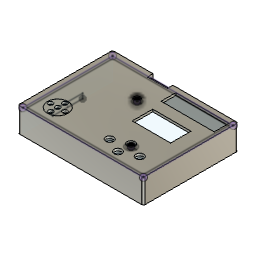
SmartDiskII 3D Case board v7 (Autodesk Fusion 360 design; units mm, degrees)
Autodesk Fusion 360 part; units mm, degrees
note: some values were not read from the file. Chosen so that the rebuilt part matches the saved one: which bodies a step acts on; which face or edge a step refers to. Set by a fixed rule: which sketch regions a step uses.
sketch "Sketch1" plane through (0, 0, 0) normal (0, 0, 1) x (1, 0, 0)
  line L0 (0, 0) -> (76.3, 0)
  line L1 (76.3, 0) -> (76.3, 56.8)
  line L2 (76.3, 56.8) -> (0, 56.8)
  line L3 (0, 56.8) -> (0, 0)
  line L4 (77.8, 58.3) -> (-1.5, 58.3)
  line L5 (-1.5, 58.3) -> (-1.5, -1.5)
  line L6 (-1.5, -1.5) -> (77.8, -1.5)
  line L7 (77.8, -1.5) -> (77.8, 58.3)
  line L8 (2.9, 56.8) -> (2.9, 58.3)
  line L9 (17.8, 56.8) -> (17.8, 58.3)
  line L10 (25.6, 56.8) -> (25.6, 58.3)
  line L11 (35.2, 58.3) -> (35.2, 56.8)
  line L12 (75.3, 58.3) -> (75.3, 56.8)
  line L13 (42.6, 58.3) -> (42.6, 56.8)
  line L14 (43.4, 38.8) -> (67.6, 38.8)
  line L15 (67.6, 38.8) -> (67.6, 25.9)
  line L16 (67.6, 25.9) -> (43.4, 25.9)
  line L17 (43.4, 25.9) -> (43.4, 38.8)
  circle A0 centre (65.2, 8.8) radius 2.5
  circle A1 centre (46.2, 8.8) radius 2.5
  circle A2 centre (55.6, 4.6) radius 2.5
  circle A3 centre (55.6, 12.9) radius 2.5
  line L18 (41.7, 55.2) -> (75.3, 55.2)
  line L19 (75.3, 55.2) -> (75.3, 45.8)
  line L20 (75.3, 45.8) -> (41.7, 45.8)
  line L21 (41.7, 45.8) -> (41.7, 55.2)
  line L22 (25.6, 56.8) -> (35.2, 56.8)
  line L23 (35.2, 56.8) -> (35.2, 47.1)
  line L24 (35.2, 47.1) -> (25.6, 47.1)
  line L25 (25.6, 47.1) -> (25.6, 56.8)
  line L26 (25.6, 42.9) -> (35.2, 42.9)
  line L27 (35.2, 42.9) -> (35.2, 36.4)
  line L28 (35.2, 36.4) -> (25.6, 36.4)
  line L29 (25.6, 36.4) -> (25.6, 42.9)
  circle A4 centre (12.4, 9.7) radius 6.5
  line L30 (25.6, 16.35) -> (30.6, 16.35)
  line L31 (30.6, 16.35) -> (30.6, 9.85)
  line L32 (30.6, 9.85) -> (25.6, 9.85)
  line L33 (25.6, 9.85) -> (25.6, 16.35)
  circle A5 centre (12, 20.2) radius 2.25
  circle A6 centre (12.4, 37.5) radius 2.25
  circle A7 centre (72.3819, 43.55) radius 1.75
  circle A8 centre (3.8963, 4.2747) radius 2.5
  circle A9 centre (72.3819, 8.8) radius 2.5
  line L34 (47.4, 40.3) -> (63.6, 40.3)
  line L35 (63.6, 40.3) -> (63.6, 44.3)
  line L36 (63.6, 44.3) -> (47.4, 44.3)
  line L37 (47.4, 44.3) -> (47.4, 40.3)
  line L38 (24.1, 58.3) -> (36.7, 58.3)
  line L39 (36.7, 58.3) -> (36.7, 56.8)
  line L40 (36.7, 56.8) -> (24.1, 56.8)
  line L41 (24.1, 56.8) -> (24.1, 58.3)
  line L42 (30.1, 42.9) -> (30.1, 36.4)
  line L43 (30.1, 36.4) -> (35.2, 42.9) construction
  line L44 (30.1, 42.9) -> (35.2, 36.4) construction
  circle A10 centre (32.65, 39.65) radius 2
  circle A11 centre (55.6, 12.9) radius 3.4
  circle A12 centre (55.6, 12.9) radius 4.15
  circle A13 centre (55.6, 4.6) radius 3.4
  circle A14 centre (55.6, 4.6) radius 4.15
  circle A15 centre (46.2, 8.8) radius 3.4
  circle A16 centre (46.2, 8.8) radius 4.15
  circle A17 centre (65.2, 8.8) radius 3.4
  circle A18 centre (65.2, 8.8) radius 4.15
  circle A19 centre (32.65, 39.65) radius 2.65
  circle A20 centre (32.65, 39.65) radius 3.4
  line L45 (12.4, 9.7) -> (12.4, 16.2) construction
  line L46 (12.4, 9.7) -> (18.9, 9.7) construction
  line L47 (12.4, 9.7) -> (12.4, 3.2) construction
  line L48 (12.4, 9.7) -> (5.9, 9.7) construction
  circle A21 centre (12.4, 9.7) radius 1.5
  circle A22 centre (12.4, 5.2) radius 1.5
  circle A23 centre (7.9, 9.7) radius 1.5
  circle A24 centre (16.9, 9.7) radius 1.5
  circle A25 centre (12.4, 14.2) radius 1.5
  dimension "d5" = 76.3
  dimension "d6" = 56.8
  dimension "d8" = 1.5
  dimension "d9" = 2.9
  dimension "d10" = 17.8
  dimension "d11" = 25.6
  dimension "d12" = 35.2
  dimension "d13" = 75.3
  dimension "d14" = 42.6
  dimension "d15" = 8.7
  dimension "d16" = 24.2
  dimension "d17" = 12.9
  dimension "d18" = 25.9
  dimension "d19" = 5
  dimension "d20" = 8.8
  dimension "d21" = 11.1
  dimension "d22" = 5
  dimension "d23" = 30.1
  dimension "d24" = 5
  dimension "d25" = 4.6
  dimension "d26" = 20.7
  dimension "d27" = 5
  dimension "d28" = 12.9
  dimension "d39" = 9.4
  dimension "d40" = 1.6
  dimension "d43" = 8.8
  dimension "d44" = 1
  dimension "d45" = 33.6
  dimension "d46" = 20.7
  dimension "d47" = 9.7
  dimension "d48" = 6.5
  dimension "d50" = 13.9
  dimension "d53" = 13
  dimension "d54" = 12.4
  dimension "d55" = 9.7
  dimension "d58" = 9.85
  dimension "d59" = 6.5
  dimension "d60" = 5
  dimension "d67" = 4.5
  dimension "d68" = 4.5
  dimension "d69" = 19.3
  dimension "d70" = 20.2
  dimension "d71" = 3.5
  dimension "d72" = 5
  dimension "d73" = 13.25
  dimension "d74" = 5
  dimension "d86" = 4
  dimension "d87" = 4
  dimension "d88" = 1.5
  dimension "d89" = 1.5
  dimension "d92" = 12.6
  dimension "d93" = 1.5
  dimension "d94" = 1.5
  dimension "d113" = 4.5
  dimension "d135" = 4
  dimension "d202" = 6.8
  dimension "d203" = 8.3
  dimension "d204" = 6.8
  dimension "d205" = 8.3
  dimension "d206" = 6.8
  dimension "d207" = 8.3
  dimension "d208" = 6.8
  dimension "d209" = 8.3
  dimension "d212" = 5.3
  dimension "d213" = 6.8
  dimension "d217" = 3
  dimension "d218" = 3
  dimension "d219" = 2
  dimension "d220" = 3
  dimension "d221" = 2
  dimension "d222" = 3
  dimension "d223" = 2
  dimension "d224" = 3
  dimension "d225" = 2
  dimension "d228" = 12
  constraint horizontal L0
  constraint vertical L1
  constraint horizontal L2
  constraint vertical L3
  constraint coincident L0.start L3.end
  constraint coincident L2 L8.start
  constraint coincident L4 L8.end
  constraint perpendicular L4 L8
  constraint coincident L2 L9.start
  constraint coincident L4 L9.end
  constraint perpendicular L4 L9
  constraint coincident L2 L10.start
  constraint coincident L4 L10.end
  constraint perpendicular L4 L10
  constraint coincident L4 L11.start
  constraint coincident L2 L11.end
  constraint perpendicular L2 L11
  constraint coincident L4 L12.start
  constraint coincident L2 L12.end
  constraint perpendicular L2 L12
  constraint coincident L4 L13.start
  constraint coincident L2 L13.end
  constraint perpendicular L2 L13
  constraint horizontal L14
  constraint vertical L15
  constraint horizontal L16
  constraint vertical L17
  constraint horizontal L18
  constraint vertical L19
  constraint horizontal L20
  constraint vertical L21
  constraint horizontal L22
  constraint vertical L23
  constraint horizontal L24
  constraint vertical L25
  constraint horizontal L26
  constraint vertical L27
  constraint horizontal L28
  constraint vertical L29
  constraint horizontal L30
  constraint vertical L31
  constraint horizontal L32
  constraint vertical L33
  constraint collinear L29 L33
  constraint horizontal L34
  constraint vertical L35
  constraint horizontal L36
  constraint vertical L37
  constraint horizontal L38
  constraint vertical L39
  constraint horizontal L40
  constraint vertical L41
  constraint coincident L4 L38.start
  constraint coincident L26 L42.start
  constraint coincident L28 L42.end
  constraint perpendicular L28 L42
  constraint midpoint L44 A10.centre
  constraint concentric A3 A11
  constraint concentric A3 A12
  constraint concentric A2 A13
  constraint concentric A13 A14
  constraint concentric A1 A15
  constraint concentric A1 A16
  constraint concentric A0 A17
  constraint concentric A0 A18
  constraint concentric A10 A19
  constraint concentric A10 A20
  constraint coincident A4.centre L45.start
  constraint coincident A4 L45.end
  constraint vertical L45
  constraint coincident A4 L46.end
  constraint perpendicular L45 L46
  constraint coincident A4 L47.end
  constraint perpendicular L46 L47
  constraint coincident A4 L48.end
  constraint perpendicular L47 L48
  constraint concentric A4 A21
  constraint coincident L47 A22.centre
  constraint coincident L48 A23.centre
  constraint coincident L46 A24.centre
  constraint coincident L45 A25.centre
  measures "d5" distance of L0.start L0.end
  measures "d6" distance of L0.start L2.end
  measures "d9" distance of L3 L8
  measures "d10" distance of L3 L9
  measures "d11" distance of L3 L10
  measures "d12" distance of L3 L11
  measures "d13" distance of L3 L12
  measures "d14" distance of L3 L13
  measures "d15" distance of L1 L15
  measures "d16" distance of L15 L17
  measures "d17" distance of L14 L16
  measures "d18" distance of L0 L16
  measures "d19" diameter of A0
  measures "d20" distance of L0 A0.centre
  measures "d21" distance of L1 A0.centre
  measures "d22" diameter of A1
  measures "d23" distance of L1 A1.centre
  measures "d24" diameter of A2
  measures "d25" distance of L0 A2.centre
  measures "d26" distance of L1 A2.centre
  measures "d27" diameter of A3
  measures "d28" distance of L0 A3.centre
  measures "d39" distance of L18.start L20.end
  measures "d40" distance of L2 L18
  measures "d43" distance of L0 A1.centre
  measures "d44" distance of L1 L19
  measures "d45" distance of L19 L21
  measures "d46" distance of L1 A3.centre
  measures "d47" distance of L10.start L24.end
  measures "d48" distance of L26.start L28.end
  measures "d50" distance of L2 L26
  measures "d53" diameter of A4
  measures "d54" distance of L3 A4.centre
  measures "d55" distance of L0 A4.centre
  measures "d58" distance of L0 L32
  measures "d59" distance of L30 L32
  measures "d60" distance of L31 L33
  measures "d67" diameter of A5
  measures "d68" diameter of A6
  measures "d69" distance of L2 A6.centre
  measures "d70" distance of L0 A5.centre
  measures "d71" diameter of A7
  measures "d72" diameter of A8
  measures "d73" distance of L2 A7.centre
  measures "d74" diameter of A9
  measures "d86" distance of L17 L37
  measures "d87" distance of L15 L35
  measures "d88" distance of L20 L36
  measures "d89" distance of L14 L34
  measures "d92" distance of L38.start L38.end
  measures "d93" distance of L10 L41
  measures "d94" distance of L11 L39
  measures "d113" distance of L29 L42
  measures "d135" diameter of A10
  measures "d202" diameter of A11
  measures "d203" diameter of A12
  measures "d204" diameter of A13
  measures "d205" diameter of A14
  measures "d206" diameter of A15
  measures "d207" diameter of A16
  measures "d208" diameter of A17
  measures "d209" diameter of A18
  measures "d212" diameter of A19
  measures "d213" diameter of A20
  measures "d217" diameter of A21
  measures "d218" diameter of A22
  measures "d219" distance of L47.end A22.centre
  measures "d220" diameter of A23
  measures "d221" distance of L48.end A23.centre
  measures "d222" diameter of A24
  measures "d223" distance of L46.end A24.centre
  measures "d224" diameter of A25
  measures "d225" distance of L45.end A25.centre
  measures "d228" distance of L3 A5.centre
extrude "Extrude1" add sketch "Sketch1" along normal blind 1.5 contours L0 L1 L2 L3 L23 L24 L25 L40 | L2 L22 L23 L24 L25 L40 | L18 L19 L20 L21 | L26 L28 L29 L42 A20 | L26 L42 A20 | L26 A20 | L26 L27 L42 A19 A20 | L42 A19 A20 | L28 L42 A20 | L26 L27 A20 | L27 L42 A19 | L42 A19 | L27 L28 L42 A19 A20 | L28 A20 | L27 A19 A20 | L27 A19 | L27 L28 A20 | A4 | L30 L31 L32 L33 | A5 | A6 | A7 | A8 | A9 | L34 L35 L36 L37 | A10 | A11 | A12 | A14 | A13 | A15 | A16 | A17 | A18 | A21 | A22 | A23 | A24 | A25 makes body 1
extrude "Extrude2" add sketch "Sketch1" against normal blind 10 contours L0 L1 L2 L3 L4 L5 L6 L7 L8 L12 | L2 L4 L12 L13 | L2 L4 L9 L41 | L2 L4 L13 L39 | L2 L4 L10 L38 L40 L41 | L2 L4 L11 L38 L39 L40 bodies 1
extrude "Extrude3" add sketch "Sketch1" along normal blind 1.5 separate body contours L0 L1 L2 L3 L4 L5 L6 L7 L8 L12 | L2 L4 L8 L9 | L2 L4 L12 L13 | L2 L4 L9 L41 | L2 L4 L13 L39 | L2 L4 L10 L38 L40 L41 | L2 L4 L11 L38 L39 L40 | L2 L4 L10 L11 L22 L38 L40 makes body 2
extrude "Extrude4" cut sketch "Sketch1" along normal blind 1.5 contours L18 L19 L20 L21 bodies 1
extrude "Extrude5" cut sketch "Sketch1" along normal blind 3 contours L2 L4 L10 L11 L22 L38 L40 | L2 L22 L23 L24 L25 L40 | L26 L28 L29 L42 A20 | L26 L42 A20 | L26 L27 L42 A19 A20 | L42 A19 A20 | L28 L42 A20 | L26 L27 A20 | L27 L42 A19 | L42 A19 | L27 L28 L42 A19 A20 | L27 L28 A20 | A4 | L30 L31 L32 L33 | A10 | A21 | A22 | A23 | A24 | A25 bodies 1 2
sketch "Sketch2" plane through (0, 0, 0) normal (0, 0, 1) x (1, 0, 0)
  circle A0 centre (55.6, 12.9) radius 2.35
  circle A1 centre (55.6, 12.9) radius 3.25
  line L0 (1.5, 1.5) -> (74.8, 1.5)
  line L1 (74.8, 1.5) -> (74.8, 55.3)
  line L2 (74.8, 55.3) -> (1.5, 55.3)
  line L3 (1.5, 55.3) -> (1.5, 1.5)
  line L4 (0, 56.8) -> (0, 0)
  line L5 (0, 0) -> (76.3, 0)
  line L6 (76.3, 0) -> (76.3, 56.8)
  line L7 (76.3, 56.8) -> (0, 56.8)
  line L8 (76.2, 0.1) -> (0.1, 0.1)
  line L9 (0.1, 0.1) -> (0.1, 56.7)
  line L10 (0.1, 56.7) -> (76.2, 56.7)
  line L11 (76.2, 56.7) -> (76.2, 0.1)
  circle A2 centre (32.65, 39.65) radius 2.5
  circle A3 centre (32.65, 39.65) radius 1.75
  point P0 (55.6, 12.9)
  point P1 (32.65, 39.65)
  dimension "d61" = 4.7
  dimension "d62" = 6.5
  dimension "d101" = 1.5
  dimension "d102" = 1.5
  dimension "d103" = 1.5
  dimension "d104" = 1.5
  dimension "d121" = 0.1
  dimension "d122" = 0.1
  dimension "d123" = 0.1
  dimension "d124" = 0.1
  dimension "d136" = 5
  dimension "d137" = 3.5
  constraint coincident P0 A0.centre
  constraint horizontal L0
  constraint vertical L1
  constraint horizontal L2
  constraint vertical L3
  constraint horizontal L8
  constraint vertical L9
  constraint horizontal L10
  constraint vertical L11
  constraint coincident P1 A2.centre
  constraint concentric A2 A3
  measures "d61" diameter of A0
  measures "d62" diameter of A1
  measures "d101" distance of L3 L4
  measures "d102" distance of L0 L5
  measures "d103" distance of L1 L6
  measures "d104" distance of L2 L7
  measures "d121" distance of L7 L10
  measures "d122" distance of L6 L11
  measures "d123" distance of L5 L8
  measures "d124" distance of L4 L9
  measures "d136" diameter of A2
  measures "d137" diameter of A3
extrude "Extrude7" add sketch "Sketch2" along normal blind 1.7 separate body contours A1 makes body 3
extrude "Extrude8" add sketch "Sketch2" along normal blind 4 contours A0 bodies 3
extrude "Extrude9" add sketch "Sketch1" against normal blind 6.9 separate body contours A5 | A6 | A7 | A8 | A9 makes body 4 at (6.3932, 4.15, -4.6) makes body 5 at (14.6472, 37.3878, -4.6) makes body 6 at (73.9944, 42.8702, -4.6) makes body 7 at (14.2472, 20.0878, -4.6) makes body 8 at (74.8788, 8.6754, -4.6)
combine "Combine1" operation add target body 4 tool bodies 7 5 6 8 makes body 9 at (14.2472, 20.0878, -4.6) makes body 10 at (73.9944, 42.8702, -4.6) makes body 11 at (14.6472, 37.3878, -4.6) makes body 12 at (74.8788, 8.6754, -4.6)
extrude "Extrude10" add sketch "Sketch1" against normal blind 5 contours L2 L4 L8 L9 bodies 1 3 2
extrude "Extrude11" add 2 faces at (25.4333, -1, -10) (23, 57.3, -10) along direction (0, 0, -1) blind 4 on bodies 1 bodies 1
extrude "Extrude12" add sketch "Sketch1" along normal blind 0.75 from surface at 0.75 contours L2 L22 L23 L24 L25 L40 | L30 L31 L32 L33 bodies 1
extrude "Extrude13" cut 1 faces at (32, 56.8, 1) along direction (0, -1, 0) blind 2 on bodies 1 bodies 1
extrude "Extrude14" cut sketch "Sketch1" along normal blind 0.75 contours L34 L35 L36 L37 bodies 1
extrude "Extrude15" cut sketch "Sketch1" along normal blind 1.5 contours L2 L4 L10 L38 L40 L41 | L2 L4 L11 L38 L39 L40 bodies 1
extrude "Extrude16" cut 2 faces at (36.2, 56.8, 0.5) (25.1, 56.8, 1) along direction (0, 1, 0) up to surface end surface through (35.2, 54.8, 0.75) normal (0, 1, 0) offset 0 on bodies 1 bodies 1
extrude "Extrude17" cut sketch "Sketch1" against normal blind 4 contours L2 L4 L10 L38 L40 L41 | L2 L4 L11 L38 L39 L40 bodies 1
fillet "Fillet1" radius 2 1 edges at (24.1, 57.55, -4) on bodies 1
fillet "Fillet1" radius 2 1 edges at (36.7, 57.55, -4) on bodies 1
extrude "Extrude18" add sketch "Sketch1" sketch "Sketch2" along normal blind 1.5 separate body contours L0 L1 L2 L3 L4 L5 L6 L7 L8 L12 | L2 L4 L8 L9 | L2 L4 L12 L13 | L2 L4 L9 L41 | L2 L4 L13 L39 | L2 L4 L10 L38 L40 L41 | L2 L4 L11 L38 L39 L40 | L2 L4 L10 L11 L22 L38 L40 of sketch 2 contours A0 | A1 | L0 L1 L2 L3 | L4 L5 L6 L7 | L8 L9 L10 L11 | A2 | A3 makes body 13
extrude "Extrude19" add sketch "Sketch2" along normal blind 6.7 contours L8 L9 L10 L11 bodies 13
extrude "Extrude20" add sketch "Sketch1" along normal blind 8.6 contours L2 L4 L8 L9 bodies 13
extrude "Extrude21" add sketch "Sketch1" along normal blind 9.5 contours L2 L4 L10 L11 L22 L38 L40 bodies 13
extrude "Extrude22" add sketch "Sketch1" along normal blind 0.75 from surface at 0.75 contours L26 L28 L29 L42 A20 | L42 A19 A20 | L42 A19 bodies 1
extrude "Extrude23" add 1 faces at (28.8, 57.8, 9.5) along direction (0, 0, 1) blind 2 on bodies 13 bodies 13
extrude "Extrude24" cut 1 faces at (25.6, 57.8, 8.1667) along direction (1, 0, 0) blind 0.1 on bodies 13 bodies 13
extrude "Extrude25" cut 1 faces at (2.9, 57.8, 6.2333) along direction (1, 0, 0) blind 0.1 on bodies 13 bodies 13
extrude "Extrude26" cut 1 faces at (17.8, 57.8, 6.2333) along direction (-1, 0, 0) blind 0.1 on bodies 13 bodies 13
extrude "Extrude27" cut 1 faces at (35.2, 57.8, 4.8333) along direction (-1, 0, 0) blind 0.1 on bodies 13 bodies 13
extrude "Extrude28" add sketch "Sketch2" along normal blind 0.5 separate body contours A2 makes body 14
extrude "Extrude29" add sketch "Sketch2" along normal blind 1.75 contours A3 bodies 14
extrude "Extrude30" add sketch "Sketch1" along normal blind 0.75 from surface at 0.75 contours L26 L42 A20 | L26 L27 L42 A19 A20 | L28 L42 A20 | L26 L27 A20 | L27 L42 A19 | L27 L28 L42 A19 A20 | L27 L28 A20 bodies 1
extrude "Extrude31" add sketch "Sketch1" along normal up to surface (10 mm away) from surface at -14 separate body contours L2 L4 L10 L11 L22 L38 L40 makes body 15
extrude "Extrude32" add sketch "Sketch1" along normal blind 7.1 from surface at -14 separate body contours L2 L4 L8 L9 makes body 16
sketch "nobes" plane through (0, 0, 0) normal (1, 0, 0) x (0, 1, 0)
  line L0 (56.8, 0) -> (0, 0)
  line L1 (0, 0) -> (0, -14)
  line L2 (0, -14) -> (56.8, -14)
  line L3 (56.8, -14) -> (56.8, 0)
  line L4 (37.8667, -14) -> (18.9333, -14)
  line L5 (18.9333, -14) -> (18.9333, -11)
  line L6 (18.9333, -11) -> (37.8667, -11)
  line L7 (37.8667, -11) -> (37.8667, -14)
  line L8 (28.4, -14) -> (28.4, -11) construction
  dimension "d151" = 18.9333
  dimension "d154" = 3
  constraint horizontal L4
  constraint vertical L5
  constraint horizontal L6
  constraint vertical L7
  constraint coincident L2 L4.start
  constraint midpoint L2 L8.start
  constraint midpoint L6 L8.end
  constraint perpendicular L4 L8
  measures "d151" distance of L5 L7
  measures "d154" distance of L4 L6
extrude "Extrude33" add sketch "nobes" along normal blind 3 draft -45 contours L2 L4 L5 L6 L7 bodies 1
ref_plane "WorkPlane1" through (38.15, 28.4, -6.25) normal (-1, 0, 0) x (0, 1, 0)
mirror "Mirror1" about plane through (38.15, 28.4, -6.25) normal (-1, 0, 0) of "Extrude33"
combine "Combine2" operation add target body 1 tool bodies 4 9 10 11 12 15 16
sketch "Sketch3" plane through (0, 0, -14) normal (0, 0, -1) x (1, 0, 0) in component "couvercle"
  line L0 (76.3, -56.8) -> (0, -56.8)
  line L1 (0, -56.8) -> (0, -37.8667)
  line L2 (0, -37.8667) -> (0, -18.9333)
  line L3 (0, -18.9333) -> (0, 0)
  line L4 (0, 0) -> (76.3, 0)
  line L5 (76.3, 0) -> (76.3, -18.9333)
  line L6 (76.3, -18.9333) -> (76.3, -37.8667)
  line L7 (76.3, -37.8667) -> (76.3, -56.8)
  line L8 (-1.5, -58.3) -> (77.8, -58.3)
  line L9 (77.8, -58.3) -> (77.8, 1.5)
  line L10 (77.8, 1.5) -> (-1.5, 1.5)
  line L11 (-1.5, 1.5) -> (-1.5, -58.3)
  line L12 (0.2, -0.2) -> (76.1, -0.2)
  line L13 (76.1, -0.2) -> (76.1, -15.7)
  line L14 (76.1, -15.7) -> (76.1, -44.1)
  line L15 (76.1, -44.1) -> (76.1, -56.6)
  line L16 (76.1, -56.6) -> (0.2, -56.6)
  line L17 (0.2, -56.6) -> (0.2, -37.6)
  line L18 (0.2, -37.6) -> (0.2, -9.2)
  line L19 (0.2, -9.2) -> (0.2, -0.2)
  line L20 (9.5, -39.4) -> (11.5, -39.4)
  line L21 (11.5, -39.4) -> (11.5, -17.4)
  line L22 (11.5, -17.4) -> (9.5, -17.4)
  line L23 (9.5, -17.4) -> (9.5, -39.4)
  line L24 (33.2, -39.4) -> (35.2, -39.4)
  line L25 (35.2, -39.4) -> (35.2, -17.4)
  line L26 (35.2, -17.4) -> (33.2, -17.4)
  line L27 (33.2, -17.4) -> (33.2, -39.4)
  line L28 (62.8, -39.4) -> (64.8, -39.4)
  line L29 (64.8, -39.4) -> (64.8, -17.4)
  line L30 (64.8, -17.4) -> (62.8, -17.4)
  line L31 (62.8, -17.4) -> (62.8, -39.4)
  line L32 (76.3, -28.4) -> (64.8, -28.4) construction
  line L33 (76.3, -28.4) -> (35.2, -28.4) construction
  line L34 (0.2, -30.4727) -> (0.2, -30.6189) construction
  line L35 (69.8, -1.5) -> (61.8, -1.5)
  line L36 (61.8, -1.5) -> (61.8, -3.5)
  line L37 (61.8, -3.5) -> (69.8, -3.5)
  line L38 (69.8, -3.5) -> (69.8, -1.5)
  dimension "d161" = 0.2
  dimension "d178" = 11
  dimension "d179" = 2
  dimension "d180" = 22
  dimension "d181" = 2
  dimension "d182" = 22
  dimension "d183" = 33
  dimension "d184" = 2
  dimension "d185" = 22
  dimension "d186" = 13
  dimension "d198" = 8
  dimension "d199" = 8
  dimension "d200" = 3
  dimension "d201" = 2
  constraint horizontal L20
  constraint vertical L21
  constraint horizontal L22
  constraint vertical L23
  constraint horizontal L24
  constraint vertical L25
  constraint horizontal L26
  constraint vertical L27
  constraint horizontal L28
  constraint vertical L29
  constraint horizontal L30
  constraint vertical L31
  constraint midpoint L6 L32.start
  constraint midpoint L29 L32.end
  constraint perpendicular L14 L32
  constraint midpoint L25 L33.end
  constraint perpendicular L14 L33
  constraint coincident L18 L34.start
  constraint coincident L18 L34.end
  constraint collinear L20 L24
  constraint horizontal L35
  constraint vertical L36
  constraint horizontal L37
  constraint vertical L38
  measures "d178" distance of L11 L23
  measures "d179" distance of L21 L23
  measures "d180" distance of L20 L22
  measures "d181" distance of L24.start L24.end
  measures "d182" distance of L24.start L26.end
  measures "d183" distance of L18 L27
  measures "d184" distance of L28.start L28.end
  measures "d185" distance of L28.start L30.end
  measures "d186" distance of L9 L29
  measures "d198" distance of L9 L38
  measures "d199" distance of L36 L38
  measures "d200" distance of L10 L35
  measures "d201" distance of L35 L37
extrude "Extrude1'" add sketch "Sketch3" along normal blind 1.5 separate body contours L0 L1 L2 L3 L4 L5 L6 L7 | L8 L9 L10 L11 | L12 L13 L14 L15 L16 L17 L18 L19 | L20 L21 L22 L23 | L24 L25 L26 L27 | L28 L29 L30 L31 | L35 L36 L37 L38 makes body 17 in component "couvercle"
extrude "Extrude2'" add sketch "Sketch3" against normal blind 3 contours L12 L13 L14 L15 L16 L17 L18 L19 | L20 L21 L22 L23 | L24 L25 L26 L27 | L28 L29 L30 L31 | L35 L36 L37 L38 bodies 17 in component "couvercle"
extrude "Extrude3'" cut sketch "nobes" along normal blind 3 draft -45 from surface at 0.2 contours L2 L4 L5 L6 L7 bodies 17 in component "couvercle"
extrude "Extrude4'" cut sketch "nobes" against normal blind 3 draft -45 from surface at 76.1 contours L2 L4 L5 L6 L7 bodies 17 in component "couvercle"
shell "Shell1" thickness 1.5 removed faces 1 at (25.5, 31.5556, -11) on bodies 17 in component "couvercle"
chamfer "Chamfer1" distance 0.6 angle 45 1 edges at (76.1, 28.4, -11) on bodies 17 in component "couvercle"
chamfer "Chamfer1" distance 0.6 angle 45 1 edges at (0.2, 28.4, -11) on bodies 17 in component "couvercle"
fillet "Fillet1'" radius 1 4 edges at (77.8, -1.5, -14.75) (77.8, 58.3, -14.75) (-1.5, 58.3, -14.75) (-1.5, -1.5, -14.75) on bodies 17 in component "couvercle"
fillet "Fillet2" radius 1 4 edges at (-1.5, -1.5, -6.25) (77.8, -1.5, -6.25) (77.8, 58.3, -6.25) (-1.5, 58.3, -6.25) on bodies 1
extrude "Extrude38" add sketch "Sketch1" along normal up to surface (1.5 mm away) separate body contours A4 makes body 18
extrude "Extrude5'" add sketch "Sketch3" against normal blind 5.25 contours L20 L21 L22 L23 | L24 L25 L26 L27 | L28 L29 L30 L31 bodies 17 in component "couvercle"
fillet "Fillet2'" radius 2 6 edges at (33.2, 28.4, -14) (62.8, 28.4, -14) (9.5, 28.4, -14) (11.5, 28.4, -14) (35.2, 28.4, -14) (64.8, 28.4, -14) on bodies 17 in component "couvercle"
extrude "Extrude34" cut 1 faces at (7.8667, 57.8, -6.9) along direction (0, 0, -1) blind 0.5 on bodies 1 bodies 1
extrude "Extrude35" add 1 faces at (7.8667, 57.8, -5) along direction (0, 0, -1) blind 0.5 on bodies 1 bodies 1
chamfer "Chamfer1'" distance 1.5 angle 45 3 edges at (10.35, 58.3, -5.5) (2.9, 58.3, -6.45) (17.8, 58.3, -6.45) on bodies 1
extrude "Extrude36" add sketch "Sketch1" against normal blind 1.8 separate body contours A12 | A14 | A16 | A18 makes body 20 at (58.9831, 12.5615, -0.6) makes body 20 at (58.9831, 4.2615, -0.6) makes body 19 at (50.3448, 8.5931, -1.2) makes body 21 at (69.3294, 8.3868, -0.6)
extrude "Extrude37" add sketch "Sketch1" against normal blind 0.5 from surface at 0.75 contours L26 L27 L42 A19 A20 | L27 L28 L42 A19 A20 bodies 1
combine "Combine3" [suppressed]
component "couvercle" placed x (1, 0, 0) y (0, 1, 0) z (0, 0, 1) at (0, 0, 0)
hidden bodies 3 13 14
equation "width = 76 mm"
equation "length = 56.5 mm"
equation "margin = 0.3 mm"
equation "d5 = width + margin"
equation "d6 = length + margin"
equation "wall_ep = 1.5 mm"
equation "d8 = wall_ep"
equation "d9 = margin + 2.6 mm"
equation "d10 = margin + 17.5 mm"
equation "d11 = margin + 25.3 mm"
equation "d12 = margin + 34.90 mm"
equation "d13 = margin + 75 mm"
equation "d14 = margin + 42.30 mm"
equation "d33 = wall_ep"
equation "d37 = wall_ep"
equation "d39 = 8.8 mm + 0.6 mm"
equation "d40 = 1.9 mm - 0.3 mm"
equation "d41 = wall_ep"
equation "d45 = 33.10 mm + 0.5 mm"
equation "d77 = -5.6 mm + 1.5 mm - 0.9 mm"
equation "d101 = wall_ep"
equation "d102 = wall_ep"
equation "d103 = wall_ep"
equation "d104 = wall_ep"
equation "d107 = 1.5 mm + 5.2 mm"
equation "d109 = 1.5 mm + 7.1 mm"
equation "d111 = 8 mm + 1.5 mm"
equation "d151 = ( length + margin ) / 3"
equation "gap = 0.20 mm"
equation "d154 = wall_ep * 2"
equation "d159 = wall_ep"
equation "d162 = -2 * wall_ep"
equation "d171 = wall_ep"
named bodies: "bouton", "couvercle", "bouton RESET", "SmallBuzzer"
